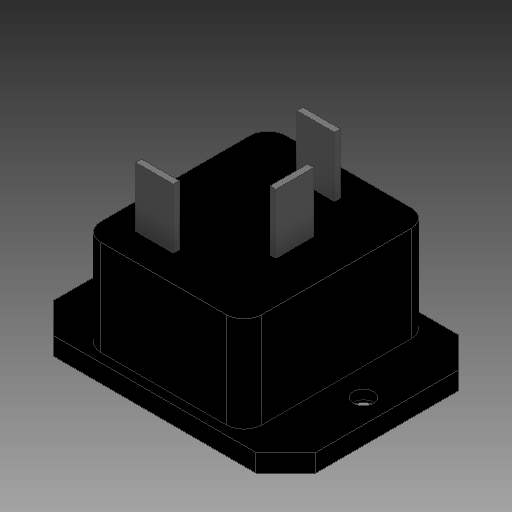
# Autodesk Inventor part: Netzstecker
Saved by Autodesk Inventor 2019 (Build 230136000, 136)
## iProperties
Created: 2018-05-16
Part Number: Netzstecker
Material: Generic
Document SubType Name: Modeling
Designer: Phil Erle
Density: 1 g/cm^3
Appearance: Default
Author: Phil Erle
Autodesk Inventor part; units mm, degrees
ref_plane "YZ Plane" through (0, 0, 0) normal (1, 0, 0) x (0, 1, 0)
ref_plane "XZ Plane" through (0, 0, 0) normal (0, 1, 0) x (-1, 0, 0)
ref_plane "XY Plane" through (0, 0, 0) normal (0, 0, 1) x (1, 0, 0)
sketch "Sketch1" plane through (0, 0, 0) normal (0, 0, 1) x (1, 0, 0)
  line L0 (-22, -17) -> (22, -17)
  line L1 (22, -17) -> (22, 17)
  line L2 (22, 17) -> (-22, 17)
  line L3 (-22, 17) -> (-22, -17)
  line L4 (-22, -17) -> (22, 17) construction
  line L5 (22, -17) -> (-22, 17) construction
  point P0 (0, 0)
  dimension "d0" = 44
  dimension "d1" = 34
  constraints: 12 end point, 2 midpoint, 2 parallel, 1 horizontal, 1 perpendicular
  measures "d0" distance of L2.end L1.end
  measures "d1" distance of L1.end L0.end
extrude "Extrusion1" add sketch "Sketch1" along normal blind 3
chamfer "Chamfer1" distance 5 angle 45 4 edges at (22, 17, 1.5) (-22, 17, 1.5) (22, -17, 1.5) (-22, -17, 1.5)
sketch "Sketch2" plane through (0, 0, 3) normal (0, 0, 1) x (1, 0, 0)
  line L0 (-13.5, -15.5) -> (13.5, -15.5)
  line L1 (13.5, -15.5) -> (13.5, 15.5)
  line L2 (13.5, 15.5) -> (-13.5, 15.5)
  line L3 (-13.5, 15.5) -> (-13.5, -15.5)
  line L4 (-13.5, -15.5) -> (13.5, 15.5) construction
  line L5 (13.5, -15.5) -> (-13.5, 15.5) construction
  point P0 (0, 0)
  dimension "d7" = 27
  dimension "d8" = 31
  constraints: 12 end point, 2 midpoint, 2 parallel, 1 horizontal, 1 perpendicular
  measures "d7" distance of L2.end L1.end
  measures "d8" distance of L1.end L0.end
extrude "Extrusion2" add sketch "Sketch2" along normal blind 16
fillet "Fillet1" radius 3 4 edges at (13.5, -15.5, 11) (13.5, 15.5, 11) (-13.5, 15.5, 11) (-13.5, -15.5, 11)
sketch "Sketch3" plane through (0, 0, 0) normal (0, 0, -1) x (-1, 0, 0)
  line L0 (-18, 0) -> (18, 0) construction
  point P0 (0, 0)
  point P1 (0, 0)
  dimension "d12" = 36
  constraints: 3 coincident, 2 end point, 1 horizontal, 1 horizontal alignment, 1 midpoint
  measures "d12" distance of L0.start L0.end
hole "Hole1" at (18, 0, 0) at (-18, 0, 0) direction (0, 0, 1) diameter 3.4 depth 8 tip angle 118 countersink diameter 6.3 countersink angle 90 clearance for "Countersunk Flat Head Screw DIN EN ISO 2009" size "M3" standard "DIN"
sketch "Sketch4" plane through (0, 0, 19) normal (0, 0, 1) x (1, 0, 0)
  line L0 (-3.15, 11) -> (3.15, 11)
  line L1 (3.15, 11) -> (3.15, 10)
  line L2 (3.15, 10) -> (-3.15, 10)
  line L3 (-3.15, 10) -> (-3.15, 11)
  line L4 (-3.15, 11) -> (3.15, 10) construction
  line L5 (3.15, 11) -> (-3.15, 10) construction
  line L6 (5.5, -3.15) -> (6.5, -3.15)
  line L7 (6.5, -3.15) -> (6.5, 3.15)
  line L8 (6.5, 3.15) -> (5.5, 3.15)
  line L9 (5.5, 3.15) -> (5.5, -3.15)
  line L10 (5.5, -3.15) -> (6.5, 3.15) construction
  line L11 (6.5, -3.15) -> (5.5, 3.15) construction
  line L12 (-9.15, -11) -> (-2.85, -11)
  line L13 (-2.85, -11) -> (-2.85, -10)
  line L14 (-2.85, -10) -> (-9.15, -10)
  line L15 (-9.15, -10) -> (-9.15, -11)
  line L16 (-9.15, -11) -> (-2.85, -10) construction
  line L17 (-2.85, -11) -> (-9.15, -10) construction
  point P0 (0, 0)
  point P1 (0, 10.5)
  point P2 (6, 0)
  point P3 (-6, -10.5)
  point P4 (0, 10.5)
  point P5 (6, 0)
  dimension "d20" = 6.3
  dimension "d21" = 1
  dimension "d22" = 1
  dimension "d23" = 6.3
  dimension "d24" = 6.3
  dimension "d25" = 1
  dimension "d26" = 10
  dimension "d27" = 6
  dimension "d28" = 10
  dimension "d29" = 6
  constraints: 36 end point, 8 midpoint, 6 parallel, 3 horizontal, 3 perpendicular, 1 horizontal alignment, 1 vertical alignment
  measures "d20" distance of L1.end L2.end
  measures "d21" distance of L0.end L1.end
  measures "d22" distance of L8.end L7.end
  measures "d23" distance of L7.end L6.end
  measures "d24" distance of L14.end L13.end
  measures "d25" distance of L13.end L12.end
  measures "d26" distance from line of point (0, 0) L2
  measures "d27" distance of point (0, 0) point (6, 0)
  measures "d28" distance from line of point (0, 0) L14
  measures "d29" horizontal distance of point (0, 0) point (-6, -10.5)
extrude "Extrusion3" add sketch "Sketch4" along normal blind 10
sketch "Sketch5" plane through (0, 0, 0) normal (0, 0, -1) x (-1, 0, 0)
  line L0 (-10, -7.5) -> (10, -7.5)
  line L1 (10, -7.5) -> (10, 7.5)
  line L2 (10, 7.5) -> (-10, 7.5)
  line L3 (-10, 7.5) -> (-10, -7.5)
  line L4 (-10, -7.5) -> (10, 7.5) construction
  line L5 (10, -7.5) -> (-10, 7.5) construction
  point P0 (0, 0)
  dimension "d32" = 20
  dimension "d33" = 15
  constraints: 12 end point, 2 midpoint, 2 parallel, 1 horizontal, 1 perpendicular
  measures "d32" distance of L2.end L1.end
  measures "d33" distance of L1.end L0.end
extrude "Extrusion4" cut sketch "Sketch5" against normal blind 10
fillet "Fillet2" radius 3 2 edges at (-10, -7.5, 5) (10, -7.5, 5)
chamfer "Chamfer2" distance 5 angle 45 2 edges at (-10, 7.5, 5) (10, 7.5, 5)
fillet "Fillet3" radius 3 4 edges at (10, 2.5, 5) (5, 7.5, 5) (-5, 7.5, 5) (-10, 2.5, 5)
sketch "Sketch6" plane through (0, 0, 10) normal (0, 0, -1) x (-1, 0, 0)
  line L0 (-1, 2) -> (1, 2)
  line L1 (1, 2) -> (1, 5.5)
  line L2 (1, 5.5) -> (-1, 5.5)
  line L3 (-1, 5.5) -> (-1, 2)
  line L4 (-6, -5.5) -> (-4, -5.5)
  line L5 (-4, -5.5) -> (-4, -2)
  line L6 (-4, -2) -> (-6, -2)
  line L7 (-6, -2) -> (-6, -5.5)
  line L8 (4, -5.5) -> (6, -5.5)
  line L9 (6, -5.5) -> (6, -2)
  line L10 (6, -2) -> (4, -2)
  line L11 (4, -2) -> (4, -5.5)
  line L12 (-4, -2) -> (4, -2) construction
  point P0 (0, 0)
  point P1 (0, 2)
  point P2 (0, -2)
  dimension "d41" = 2
  dimension "d42" = 2
  dimension "d43" = 2
  dimension "d44" = 3.5
  dimension "d45" = 3.5
  dimension "d46" = 2
  dimension "d47" = 2
  dimension "d48" = 8
  constraints: 26 end point, 6 parallel, 4 horizontal, 3 perpendicular, 2 midpoint, 2 point on line, 2 vertical alignment
  measures "d41" distance of L1.end L2.end
  measures "d42" distance of L5.end L6.end
  measures "d43" distance of L9.end L10.end
  measures "d44" distance of L8.end L9.end
  measures "d45" distance of L0.end L1.end
  measures "d46" distance of point (0, 0) point (0, 2)
  measures "d47" distance of point (0, 0) point (0, -2)
  measures "d48" distance of L5.end L10.end
extrude "Extrusion5" add sketch "Sketch6" along normal blind 8
chamfer "Chamfer3" distance 0.5 angle 45 12 edges at (5, -2, 2) (6, -3.75, 2) (4, -3.75, 2) (5, -5.5, 2) (0, 2, 2) (1, 3.75, 2) (0, 5.5, 2) (-1, 3.75, 2) (-4, -3.75, 2) (-5, -2, 2) (-6, -3.75, 2) (-5, -5.5, 2)
body "Solid1"
